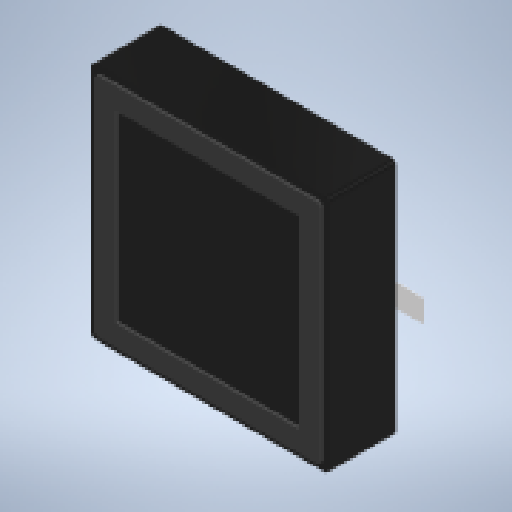
# Autodesk Inventor part: HEPA Filter
Saved by Autodesk Inventor 2024 (Build 280153000, 153)
## iProperties
Created: 2024-09-27
Part Number: HEPA Filter
Material: Generic
Document SubType Name: Modeling
Designer: Ishaan
Density: 1 g/cm^3
Appearance: Smooth - Black
Author: Ishaan
Autodesk Inventor part; units mm, degrees
ref_plane "YZ Plane" through (0, 0, 0) normal (1, 0, 0) x (0, 1, 0)
ref_plane "XZ Plane" through (0, 0, 0) normal (0, 1, 0) x (-1, 0, 0)
ref_plane "XY Plane" through (0, 0, 0) normal (0, 0, 1) x (1, 0, 0)
sketch "Sketch1" plane through (0, 0, 0) normal (0, 0, 1) x (1, 0, 0)
  line L0 (50, -50) -> (-50, -50)
  line L1 (-50, -50) -> (-50, 50)
  line L2 (-50, 50) -> (50, 50)
  line L3 (50, 50) -> (50, -50)
  line L4 (50, -50) -> (-50, 50) construction
  line L5 (-50, -50) -> (50, 50) construction
  line L6 (45.5, -47.5) -> (-45.5, -47.5)
  line L7 (-47.5, -45.5) -> (-47.5, 45.5)
  line L8 (-45.5, 47.5) -> (45.5, 47.5)
  line L9 (47.5, 45.5) -> (47.5, -45.5)
  line L10 (47.5, -47.5) -> (-47.5, 47.5) construction
  line L11 (-47.5, -47.5) -> (47.5, 47.5) construction
  line L12 (38.5, 38.5) -> (-38.5, 38.5)
  line L13 (-38.5, 38.5) -> (-38.5, -38.5)
  line L14 (-38.5, -38.5) -> (38.5, -38.5)
  line L15 (38.5, -38.5) -> (38.5, 38.5)
  arc A0 (-45.5, 47.5) -> (-47.5, 45.5) centre (-45.5, 45.5) ccw
  arc A1 (47.5, 45.5) -> (45.5, 47.5) centre (45.5, 45.5) ccw
  arc A2 (45.5, -47.5) -> (47.5, -45.5) centre (45.5, -45.5) ccw
  arc A3 (-47.5, -45.5) -> (-45.5, -47.5) centre (-45.5, -45.5) ccw
  point P0 (0, 0)
  dimension "d0" = 100
  dimension "d1" = 100
  dimension "d2" = 95
  dimension "d3" = 95
  dimension "d4" = 9
  dimension "d5" = 2
  constraints: 32 end point, 8 point on circle, 8 point on line, 8 tangent, 6 parallel, 4 centre point, 4 midpoint, 3 equal radius, 3 perpendicular, 2 horizontal, 3 other
  measures "d0" distance of L1.end L2.end
  measures "d1" distance of L0.end L1.end
  measures "d2" distance of L10.end L11.end
  measures "d3" distance of L11.start L10.end
  measures "d4" distance between parallel lines of L8 L12
  measures "d5" radius of A0
extrude "Extrusion1" add sketch "Sketch1" along normal mid plane 28 contours L0 L1 L2 L3 | L6 A3 L7 A0 L8 A1 L9 A2 | L15 L14 L13 L12
extrude "Extrusion2" add sketch "Sketch1" along normal mid plane 30.5 contours L6 A3 L7 A0 L8 A1 L9 A2
fillet "Fillet1" radius 2 4 edges at (50, 50, 0) (-50, 50, 0) (-50, -50, 0) (50, -50, 0)
sketch "Sketch2" plane through (0, 0, -15.25) normal (0, 0, -1) x (-1, 0, 0)
  line L0 (45.5, 47.5) -> (-45.5, 47.5) projected
  arc A0 (-45.5, 47.5) -> (-47.5, 45.5) centre (-45.5, 45.5) ccw projected
  line L1 (-47.5, 45.5) -> (-47.5, -45.5) projected
  arc A1 (-47.5, -45.5) -> (-45.5, -47.5) centre (-45.5, -45.5) ccw projected
  line L2 (-45.5, -47.5) -> (45.5, -47.5) projected
  arc A2 (45.5, -47.5) -> (47.5, -45.5) centre (45.5, -45.5) ccw projected
  line L3 (47.5, -45.5) -> (47.5, 45.5) projected
  arc A3 (47.5, 45.5) -> (45.5, 47.5) centre (45.5, 45.5) ccw projected
  line L4 (-38.5, -38.5) -> (-38.5, 38.5) projected
  line L5 (-38.5, 38.5) -> (38.5, 38.5) projected
  line L6 (38.5, 38.5) -> (38.5, -38.5) projected
  line L7 (38.5, -38.5) -> (-38.5, -38.5) projected
  line L8 (-60.4, 4.75) -> (-38.4, 4.75)
  line L9 (-38.4, 4.75) -> (-38.4, -4.75)
  line L10 (-38.4, -4.75) -> (-60.4, -4.75)
  line L11 (-60.4, -4.75) -> (-60.4, 4.75)
  point P0 (0, 0)
  point P1 (-47.5, -4.75)
  point P2 (-60.4, 0)
  point P3 (-47.5, 0)
  point P4 (-47.5, 4.75)
  dimension "d11" = 9.5
  dimension "d12" = 22
  dimension "d19" = 0.1
  constraints: 8 end point, 2 midpoint, 2 parallel, 1 horizontal, 1 horizontal alignment, 1 perpendicular
  measures "d11" distance between parallel lines of L10 L8
  measures "d12" distance of L8.start L8.end
  measures "d19" distance between parallel lines of L9 L4
extrude "Extrusion3" add sketch "Sketch2" along normal blind 0.001 and the other way blind 0.2 contours L8 L4 L10 L1 | L1 L10 L11 L8 | L8 L9 L10 L4
fillet "Fillet2" radius 0.5 2 edges at (38.4, 4.75, -15.1505) (38.4, -4.75, -15.1505)
equation "\"d2\" = d3"
body "Solid1"
